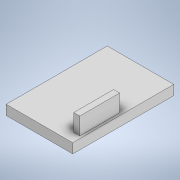
# Autodesk Inventor part: Screen_Model
Saved by Autodesk Inventor 2021 (Build 250183000, 183)
## iProperties
Created: 2020-07-08
Part Number: Screen_Model
Material: Generic
Document SubType Name: Modeling
Designer: ameli
Density: 1 g/cm^3
Appearance: Default
Author: ameli
Autodesk Inventor part; units mm, degrees
ref_plane "YZ Plane" through (0, 0, 0) normal (1, 0, 0) x (0, 1, 0)
ref_plane "XZ Plane" through (0, 0, 0) normal (0, 1, 0) x (-1, 0, 0)
ref_plane "XY Plane" through (0, 0, 0) normal (0, 0, 1) x (1, 0, 0)
sketch "Sketch1" plane through (0, 0, 0) normal (0, 1, 0) x (-1, 0, 0)
  line L0 (28, 42.5) -> (-28, 42.5)
  line L1 (-28, 42.5) -> (-28, -42.5)
  line L2 (-28, -42.5) -> (28, -42.5)
  line L3 (28, -42.5) -> (28, 42.5)
  point P0 (0, 0)
  dimension "d0" = 56
  dimension "d1" = 85
  dimension "d4" = 28
  dimension "d5" = 42.5
  constraints: 8 end point, 2 parallel, 1 horizontal, 1 perpendicular
  measures "d0" distance of L1.end L2.end
  measures "d1" distance of L2.end L0.start
  measures "d4" distance from line of point (0, 0) L3
  measures "d5" distance from line of point (0, 0) L2
extrude "Extrusion1" add sketch "Sketch1" along normal blind 8.2
sketch "Sketch3" plane through (0, 8.2, 0) normal (0, 1, 0) x (1, 0, 0)
  line L0 (20.9, -34.6) -> (26, -34.6)
  line L1 (26, -34.6) -> (26, -1.1)
  line L2 (26, -1.1) -> (20.9, -1.1)
  line L3 (20.9, -1.1) -> (20.9, -34.6)
  line L4 (-28, -42.5) -> (28, -42.5) projected
  line L5 (28, -42.5) -> (28, 42.5) projected
  point P0 (0, 0)
  dimension "d6" = 33.5
  dimension "d7" = 5.1
  dimension "d8" = 7.9
  dimension "d9" = 2
  constraints: 8 end point, 2 parallel, 1 horizontal, 1 perpendicular
  measures "d6" distance of L2.end L0.start
  measures "d7" distance of L1.end L2.end
  measures "d8" distance between parallel lines of L4 L0
  measures "d9" distance between parallel lines of L5 L1
extrude "Extrusion2" add sketch "Sketch3" along normal blind 14.5
body "Solid1"
